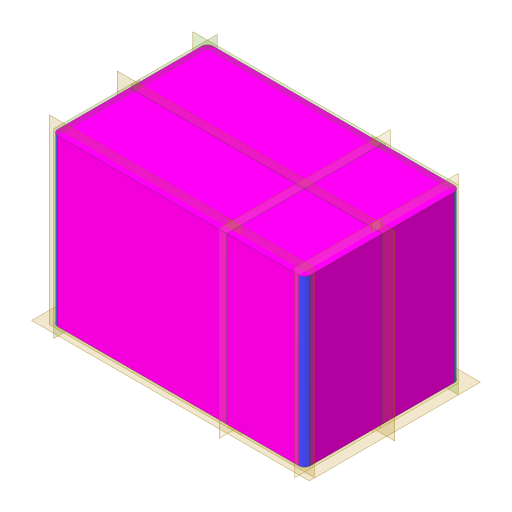
# Autodesk Inventor part: Korpus
Saved by Autodesk Inventor 2023.2 (Build 272271030, 271C)
## iProperties
Created: 2024-12-20
Part Number: Korpus
Material: Типовые
Document SubType Name: Modeling
Designer: I9232
Density: 1 g/cm^3
Appearance: По умолчанию
Author: I9232
Autodesk Inventor part; units mm, degrees
ref_plane "YZ Plane" through (0, 0, 0) normal (1, 0, 0) x (0, 1, 0)
ref_plane "XY Plane" through (0, 0, 0) normal (0, 0, 1) x (1, 0, 0)
sketch "Эскиз1" plane through (0, 0, 0) normal (0, 1, 0) x (-1, 0, 0)
  line L0 (325, 200) -> (-325, 200)
  line L1 (-325, 200) -> (-325, -200)
  line L2 (-325, -200) -> (325, -200)
  line L3 (325, -200) -> (325, 200)
  line L4 (325, 200) -> (-325, -200) construction
  line L5 (-325, 200) -> (325, -200) construction
  point P0 (0, 0)
  dimension "d0" = 650
  dimension "d1" = 400
  constraints: 12 end point, 2 midpoint, 2 parallel, 1 horizontal, 1 perpendicular
  measures "d0" distance of L1.end L2.end
  measures "d1" distance of L0.end L1.end
extrude "Выдавливание1" add sketch "Эскиз1" along normal blind 425
shell "Оболочка1" thickness 15 removed faces 0
ref_plane "РабПлоскость1" through (125, 0, 200) normal (1, 0, 0) x (0, 0, -1)
split body "Разделение1" result two bodies by plane through (125, 0, 200) normal (1, 0, 0) first body at (324.5, 141.6667, 66.6667)
ref_plane "РабПлоскость2" through (-325, 0, 0) normal (0, 0, 1) x (1, 0, 0)
split body "Разделение2" result two bodies by plane through (-325, 0, 0) normal (0, 0, 1) bodies 3 first body at (-175, 141.6667, 199.5)
split body "Разделение3" result two bodies by plane through (-325, 0, 0) normal (0, 0, 1) bodies 2 first body at (191.6667, 141.6667, 199.5)
ref_plane "РабПлоскость3" through (-310, 0, 200) normal (-1, 0, 0) x (0, 0, 1)
ref_plane "РабПлоскость4" through (-310, 0, -200) normal (-1, 0, 0) x (0, 0, 1)
ref_plane "РабПлоскость6" through (-325, 0, -185) normal (0, 0, -1) x (-1, 0, 0)
ref_plane "РабПлоскость7" through (-325, 0, 185) normal (0, 0, 1) x (1, 0, 0)
sketch "Эскиз2" plane through (0, 425, 0) normal (0, 1, 0) x (1, 0, 0)
  line L0 (-310, -280) -> (-310, 280) projected
  line L1 (455, -185) -> (-455, -185) projected
  line L2 (-325, -200) -> (125, -200) projected
  line L3 (-325, 0) -> (-325, -200) projected
  line L4 (-310, -185) -> (125, -185) projected
  arc A0 (-325, -185) -> (-310, -200) centre (-310, -185) ccw
  line L5 (125, 200) -> (-325, 200) projected
  line L6 (-325, 200) -> (-325, 0) projected
  point P0 (0, 0)
  point P1 (-310, 200)
  point P2 (-325, 185)
  constraints: 7 point on line, 2 point on circle, 1 centre point
extrude "Выдавливание2" cut sketch "Эскиз2" against normal up to surface (425 mm away) contours L2 L3 A0 bodies 4
sketch "Эскиз3" plane through (0, 425, 0) normal (0, 1, 0) x (1, 0, 0)
  line L0 (-455, 185) -> (455, 185) projected
  line L1 (-310, -280) -> (-310, 280) projected
  line L2 (125, 200) -> (-325, 200) projected
  line L3 (-325, 200) -> (-325, 0) projected
  arc A0 (-310, 200) -> (-325, 185) centre (-310, 185) ccw
  point P0 (0, 0)
  constraints: 4 point on line, 2 point on circle, 1 centre point
extrude "Выдавливание3" cut sketch "Эскиз3" against normal up to surface (425 mm away) contours L3 L2 A0 bodies 5
ref_plane "РабПлоскость8" through (310, 0, -200) normal (1, 0, 0) x (0, 0, -1)
ref_plane "РабПлоскость9" through (310, 0, 200) normal (1, 0, 0) x (0, 0, -1)
ref_plane "РабПлоскость10" through (325, 0, -185) normal (0, 0, -1) x (-1, 0, 0)
ref_plane "РабПлоскость11" through (325, 0, 185) normal (0, 0, 1) x (1, 0, 0)
sketch "Эскиз5" plane through (0, 425, 0) normal (0, 1, 0) x (1, 0, 0)
  line L0 (310, 0) -> (310, 185) projected
  line L1 (325, 200) -> (125, 200) projected
  arc A0 (325, 185) -> (310.0009, 200) centre (310, 185) ccw
  line L2 (-455.0593, 185) -> (455.3561, 185) projected
  line L3 (325, 0) -> (325, 200) projected
  line L4 (325, 200) -> (125, 200) projected
  point P0 (0, 0)
  constraints: 2 point on circle, 2 point on line, 1 centre point
extrude "Выдавливание4" cut sketch "Эскиз5" against normal up to surface (425 mm away) bodies 7
sketch "Эскиз6" plane through (0, 425, 0) normal (0, 1, 0) x (1, 0, 0)
  line L0 (455, -185) -> (-455, -185) projected
  line L1 (325, -200) -> (325, 0) projected
  line L2 (125, -200) -> (325, -200) projected
  line L3 (125, -185) -> (310, -185) projected
  line L4 (325, -200) -> (325, 0) projected
  arc A0 (310, -200) -> (325, -185) centre (310, -185) ccw
  line L5 (310, 280.0553) -> (310, -280.3319) projected
  point P0 (0, 0)
  constraints: 3 point on line, 2 point on circle, 1 centre point
extrude "Выдавливание5" cut sketch "Эскиз6" against normal up to surface (425 mm away) contours L1 L2 A0 bodies 6
